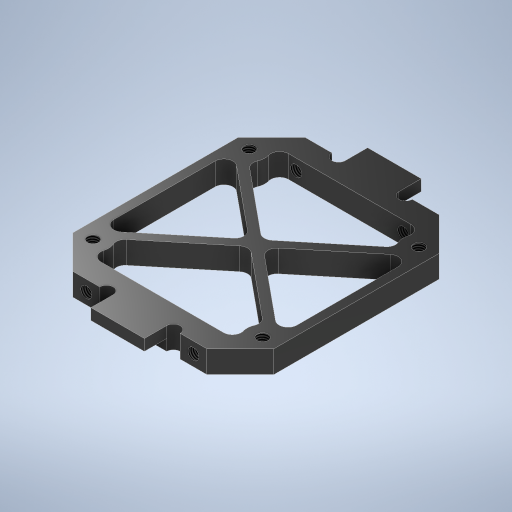
# Autodesk Inventor part: FootBraceFrame
Saved by Autodesk Inventor 2024.2 (Build 282272000, 272)
## iProperties
Created: 2024-01-07
Part Number: FootBraceFrame
Material: Aluminum 7075
Document SubType Name: Modeling
Designer: Masato Kubotera
Density: 2.81 g/cm^3
Appearance: Glossy - Black
Vendor: meviy
Mass: 11.7635 g
Surface Area: 46.1424 cm^2
Volume: 4.18629 cm^3
Author: Masato Kubotera
Autodesk Inventor part; units mm, degrees
ref_plane "YZ Plane" through (0, 0, 0) normal (1, 0, 0) x (0, 1, 0)
ref_plane "XZ Plane" through (0, 0, 0) normal (0, 1, 0) x (-1, 0, 0)
ref_plane "XY Plane" through (0, 0, 0) normal (0, 0, 1) x (1, 0, 0)
sketch "Sketch1" plane through (0, 0, 0) normal (0, 0, 1) x (1, 0, 0)
  line L0 (-31, 22.5) -> (31, 22.5)
  line L1 (31, 22.5) -> (31, -22.5)
  line L2 (31, -22.5) -> (-31, -22.5)
  line L3 (-31, -22.5) -> (-31, 22.5)
  line L4 (-31, 22.5) -> (31, -22.5) construction
  line L5 (31, 22.5) -> (-31, -22.5) construction
  line L6 (31, -6) -> (26, -6)
  line L7 (26, -6) -> (26, -15)
  line L8 (26, -15) -> (18.5, -22.5)
  line L9 (0, -22.5) -> (0, 22.5)
  line L10 (-31, 0) -> (31, 0) construction
  line L11 (31, 6) -> (26, 6)
  line L12 (26, 6) -> (26, 15)
  line L13 (26, 15) -> (18.5, 22.5)
  arc A0 (26, 9) -> (26, 6) centre (26, 7.5) ccw
  line L14 (26, 12) -> (20, 12) construction
  arc A1 (26, -6) -> (26, -9) centre (26, -7.5) ccw
  line L15 (26, -12) -> (20, -12) construction
  circle A2 centre (17.5, 19) radius 1.5 construction
  line L16 (20, 10.5) -> (20, 13.5) construction
  line L17 (-31, 22.5) -> (-31, -22.5)
  line L18 (-31, -6) -> (-26, -6)
  line L19 (-26, -6) -> (-26, -15)
  line L20 (-26, -15) -> (-18.5, -22.5)
  line L21 (-26, 15) -> (-18.5, 22.5)
  line L22 (-26, 6) -> (-26, 15)
  line L23 (-31, 6) -> (-26, 6)
  arc A3 (-26, 6) -> (-26, 9) centre (-26, 7.5) ccw
  arc A4 (-26, -9) -> (-26, -6) centre (-26, -7.5) ccw
  line L24 (-18.5, -22.5) -> (18.5, 22.5) construction
  line L25 (18.5, -22.5) -> (-18.5, 22.5) construction
  line L26 (2.339, 1.2702) -> (13.8005, 15.2098)
  line L27 (21, -13.7085) -> (21, 13.7085)
  arc A5 (16.1289, 15.7798) -> (18.4545, 15.6327) centre (17.5, 19) ccw
  line L28 (-12.8721, 17.2298) -> (-1.5449, 3.4534)
  line L29 (12.8721, 17.2298) -> (1.5449, 3.4534)
  line L30 (-11.3272, 20.5) -> (11.3272, 20.5)
  line L31 (2.339, -1.2702) -> (13.8005, -15.2098)
  arc A6 (18.4545, -15.6327) -> (16.1289, -15.7798) centre (17.5, -19) ccw
  arc A7 (21, 13.7085) -> (18.4545, 15.6327) centre (19, 13.7085) ccw
  arc A8 (16.1289, 15.7798) -> (13.8005, 15.2098) centre (15.3453, 13.9396) ccw
  arc A9 (2.339, 1.2702) -> (2.339, -1.2702) centre (3.8839, 0) ccw
  arc A10 (13.8005, -15.2098) -> (16.1289, -15.7798) centre (15.3453, -13.9396) ccw
  arc A11 (18.4545, -15.6327) -> (21, -13.7085) centre (19, -13.7085) ccw
  arc A12 (12.8721, 17.2298) -> (11.3272, 20.5) centre (11.3272, 18.5) ccw
  arc A13 (-1.5449, 3.4534) -> (1.5449, 3.4534) centre (0, 4.7236) ccw
  arc A14 (-11.3272, 20.5) -> (-12.8721, 17.2298) centre (-11.3272, 18.5) ccw
  line L32 (-12.8721, -17.2298) -> (-1.5449, -3.4534)
  line L33 (12.8721, -17.2298) -> (1.5449, -3.4534)
  line L34 (-11.3272, -20.5) -> (11.3272, -20.5)
  arc A15 (11.3272, -20.5) -> (12.8721, -17.2298) centre (11.3272, -18.5) ccw
  arc A16 (1.5449, -3.4534) -> (-1.5449, -3.4534) centre (0, -4.7236) ccw
  arc A17 (-12.8721, -17.2298) -> (-11.3272, -20.5) centre (-11.3272, -18.5) ccw
  line L35 (26, -6) -> (26, 6)
  arc A18 (18.4545, 15.6327) -> (16.1289, 15.7798) centre (17.5, 19) ccw construction
  point P0 (0, 0)
  point P1 (-17.5, 19)
  point P2 (-17.5, 19)
  point P3 (-17.5, -19)
  point P4 (-17.5, -19)
  point P5 (1.2946, 0)
  point P6 (14.9477, 16.6051)
  point P7 (21, 19)
  point P8 (0, 1.5745)
  point P9 (14.9477, -16.6051)
  point P10 (21, -19)
  point P11 (0, 2.7236)
  point P12 (0, -2.7236)
  point P13 (0, -20.5)
  point P14 (26, -9)
  point P15 (0, 20.5)
  dimension "d0" = 62
  dimension "d1" = 45
  dimension "d2" = 1.5
  dimension "d3" = 12
  dimension "d4" = 5
  dimension "d5" = 30
  dimension "d6" = 6
  dimension "d7" = 3
  dimension "d8" = 3
  dimension "d10" = 2
  dimension "d11" = 2
  dimension "d12" = 5
  dimension "d13" = 45
  dimension "d14" = 2
  dimension "d36" = 38
  dimension "d37" = 35
  dimension "d38" = 2
  constraints: 72 end point, 40 point on circle, 39 symmetric about line, 19 centre point, 18 point on line, 18 tangent, 7 equal radius, 7 midpoint, 6 coincident, 4 horizontal, 3 parallel, 2 perpendicular, 2 vertical, 9 other
  measures "d0" distance of L1.end L2.end
  measures "d1" distance of L0.end L1.end
  measures "d2" radius of A0
  measures "d3" distance between parallel lines of L11 L6
  measures "d4" distance of L11.start L12.start
  measures "d5" distance of L7.end L13.start
  measures "d6" distance of L14.end L14.start
  measures "d7" diameter of A2
  measures "d8" distance of L16.start L16.end
  measures "d10" distance between parallel lines of L0 L30
  measures "d11" distance between parallel lines of L26 L29
  measures "d12" distance between parallel lines of L12 L27
  measures "d13" angle of L12 L13
  measures "d14" radius of A7
  measures "d36" distance of point (17.5, 19) point (17.5, -19)
  measures "d37" distance of A2.centre point (-17.5, 19)
  measures "d38" radial gap between concentric circles of A2 A18
extrude "Extrusion1" add sketch "Sketch1" along normal blind 5 contours L0 L13 L12 A0 L35 A1 L7 L8 L2 L9 L34 A15 L33 A16 A13 L29 A12 L30 | L1 L6 L35 L11
extrude "Extrusion2" cut sketch "Sketch1" along normal blind 2.5 contours L1 L6 L35 L11
sketch "Sketch2" plane through (26, -6, 0) normal (1, 0, 0) x (0, 0, -1)
  line L0 (0, -6) -> (-5, -6) construction
  line L1 (-5, -9) -> (-5, -3) projected
  line L2 (0, 18) -> (-5, 18) construction
  line L3 (-5, 15) -> (-5, 21) projected
  point P0 (0, 6)
  point P1 (-2.5, -6)
  point P2 (-2.5, 18)
  constraints: 4 end point, 4 midpoint, 2 horizontal
hole "Hole1" at (26, -12, 2.5) at (26, 12, 2.5) direction (-1, 0, 0) diameter 2.459 depth 6 thread size "M3x0.5" class "6H" standard "ANSI Metric M Profile"
hole "Hole2" at (17.5, -19, 0) at (17.5, 19, 0) direction (0, 0, 1) diameter 2.459 end through all thread size "M3x0.5" class "6H" standard "ANSI Metric M Profile"
mirror "Mirror1" about plane through (0, 2.7236, 0) normal (-1, 0, 0)
equation "\"d11\" = d10"
body "Solid1"
